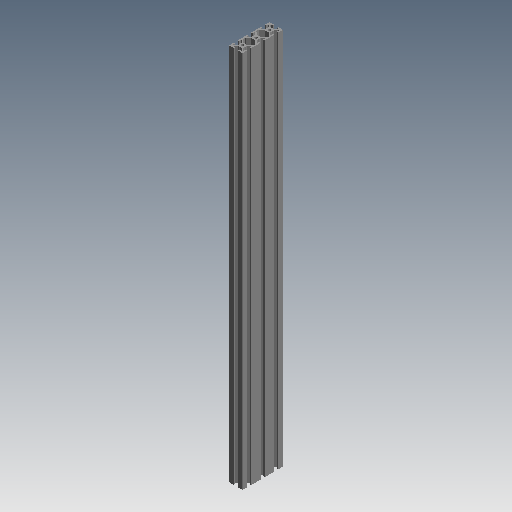
# Autodesk Inventor part: HFS5-2060-560
Saved by Autodesk Inventor 2020.1 (Build 241239000, 239)
## iProperties
Part Number: HFS5-2060-560
Material: 一般
Catalog Web Link: www.cadenas.de
Description: HFS5-2060, HFS5-2080, HFS5-4060, HFS5-4080, NFS5-2060, NFS5-2080, NFS5-4060, NFS5-4080-HFS5 Series Aluminum Extrusions 20mm Square -3 or more slots-
Vendor: MISUMI
Document SubType Name: Modeling
Designer: partserver
Manufacturer: MISUMI
Mass: 260.52 g
Surface Area: 2561.35 cm^2
Volume: 260.52 cm^3
Density: 1 g/cm^3
Appearance: PSOLRGB-175-175-175
Category: PARTsolutions
Company: MISUMI
PSOL_IDENT_0: {$CADENAS_DATA\23d-libs\misumi\metric\38_al_extrusions_blackets\5\hfs5_2060.prj},622 {VTYP=3D},{NB=H
PSOL_IDENT_1: FS5-2060-560},{LINA=HFS5-2060-560},{NN=HFS5-2060, HFS5-2080, HFS5-4060, HFS5-4080, NFS5-2060, NFS5-2
PSOL_IDENT_2: 080, NFS5-4060, NFS5-4080},{DATE=09.09.2019 15:28:27},{GEOMDATE=24.05.2018 01:50:00},{VERSION=},{LIN
PSOL_IDENT_3: EID=150},{WBVAR=L,ALT1,ALT2,ALT4,ALT5,CP5,DL5,DR5,ALT6,ALT9,ALT10,ALT11,HP6,NHL6,DL6,NHR6,DR6,ALT7,A
PSOL_IDENT_4: LT8,NH9,AH,BH,CH,DH,EH,NH10,AV,BV,CV,DV,EV,NH11,AP,BP,CP,DP,EP,ALT12,ALT13,Z,NH12,XA,XB,XC,XD,XE,NH1
PSOL_IDENT_5: 3,YA,YB,YC,YD,YE,ALT16,HP16,DL16,DR16,ALT17,HQ17,JLP,ALT18,HQ18,KLP,ALT20},{WBNUMERIC=L,NH9,AH,BH,CH
PSOL_IDENT_6: ,DH,EH,NH10,AV,BV,CV,DV,EV,NH11,AP,BP,CP,DP,EP,NH12,XA,XB,XC,XD,XE,NH13,YA,YB,YC,YD,YE,HQ17,JLP,HQ18
PSOL_IDENT_7: ,KLP}  {NB=HFS5-2060-560},{LINA=HFS5-2060-560},{KT=DUMMY},{PN=HFS5-2060-560},{TPS=HFS5-2060},{MAT=A6
PSOL_IDENT_8: N01SS-T5 Aluminum Alloy},{ST=Clear Anodize},{FRMW=20},{FRMH=60},{FRD=4.2},{L=560},{MASS=1.26},{SA=46
PSOL_IDENT_9: 4},{LX=1.97x10^4},{LY=15.98x10^4},{ALT1=},{M1=0},{DPL1=0},{DPR1=0},{ALT1PN=},{ALT2=},{ALT2ALG= '','w
PSOL_IDENT_10: /o End Tapping (Heli-Coil Insert)','LHP','with LHP (Tapping on the Left (Heli-Coil Insert))','RHP','
PSOL_IDENT_11: with RHP (Tapping on the Right (Heli-Coil Insert))','HPW','with HPW (Tapping on Both Ends (Heli-Coil
PSOL_IDENT_12: Insert))' },{M2=0},{DP2=0},{ALT2PN=},{ALT4=},{ALT4ALG= '', 'w/o SC (High Precision Cut)', 'SC', 'wi
PSOL_IDENT_13: th SC (High Precision Cut)' },{ALT4PN=},{ALT5=},{ALT5ALG= '','w/o 45 Degree Cut','1','with 45 Degree
PSOL_IDENT_14: Cut' },{CP5=},{CP5ALG= '','N/A' },{DL5=},{DL5ALG= '','N/A' },{DR5=},{DR5ALG= '','N/A' },{FRMLALT5=0
PSOL_IDENT_15: },{FRMRALT5=0},{ALT5PN=},{ALT6=},{ALT6ALG= '','w/o Fastening Location Wrench Access Hole Alterations'
PSOL_IDENT_16: ,'1','with Fastening Location Wrench Access Hole Alterations' },{ALT9=},{ALT9ALG= '','w/o Location S
PSOL_IDENT_17: pecified Wrench Access Hole Alteratons (Horizontal)','1','with Location Specified Wrench Access Hole
PSOL_IDENT_18: Alteratons (Horizontal)' },{ALT10=},{ALT10ALG= '','w/o Location Specified Wrench Access Hole Altera
PSOL_IDENT_19: tons (Vertical)','1','with Location Specified Wrench Access Hole Alteratons (Vertical)' },{ALT11=},{
PSOL_IDENT_20: ALT11ALG= '','w/o Location Specified Wrench Access Hole Alteratons (Crisscross)','1','with Location
PSOL_IDENT_21: Specified Wrench Access Hole Alteratons (Crisscross)' },{DD6=0.00},{DD6ALG=0},{HP6=},{HP6ALG= '','N/
PSOL_IDENT_22: A' },{NHL6=},{NHL6ALG= '','N/A' },{DL6=},{DL6ALG= '','N/A' },{NHR6=},{NHR6ALG= '','N/A' },{DR6=},{DR
PSOL_IDENT_23: 6ALG= '','N/A' },{DD6PN=},{HL6=0},{HL6D=0},{HR6=0},{HR6D=0},{J6=0},{J6D=0},{K6=0},{K6D=0},{ALT7=},{A
PSOL_IDENT_24: LT7ALG= '','N/A' },{ALT8=},{ALT8ALG= '','N/A' },{ALT678PN=},{NH9=0},{NH9MAX=5},{NH9ALG=[0]},{AH=0.0}
PSOL_IDENT_25: ,{AHMIN=7},{AHMAX=555},{AHALG=[0]},{BH=0.0},{BHMIN=2},{BHMAX=557},{BHALG=[0]},{CH=0.0},{CHMIN=2},{CH
PSOL_IDENT_26: MAX=559},{CHALG=[0]},{DH=0.0},{DHMIN=2},{DHMAX=561},{DHALG=[0]},{EH=0.0},{EHMIN=2},{EHMAX=553},{EHAL
PSOL_IDENT_27: G=[0]},{NH10=0},{NH10MAX=5},{NH10ALG=[0]},{AV=0.0},{AVMIN=7},{AVMAX=555},{AVALG=[0]},{BV=0.0},{BVMIN=
PSOL_IDENT_28: 2},{BVMAX=557},{BVALG=[0]},{CV=0.0},{CVMIN=2},{CVMAX=559},{CVALG=[0]},{DV=0.0},{DVMIN=2},{DVMAX=561}
PSOL_IDENT_29: ,{DVALG=[0]},{EV=0.0},{EVMIN=2},{EVMAX=553},{EVALG=[0]},{NH11=0},{NH11MAX=5},{NH11ALG=[0]},{AP=0.0},
PSOL_IDENT_30: {APMIN=7},{APMAX=555},{APALG=[0]},{BP=0.0},{BPMIN=2},{BPMAX=557},{BPALG=[0]},{CP=0.0},{CPMIN=2},{CPM
PSOL_IDENT_31: AX=559},{CPALG=[0]},{DP=0.0},{DPMIN=2},{DPMAX=561},{DPALG=[0]},{EP=0.0},{EPMIN=2},{EPMAX=553},{EPALG=
PSOL_IDENT_32: [0]},{ALT9PN=},{ALT10PN=},{ALT11PN=},{ALT91011PN=},{ALT12=},{ALT12ALG= '','w/o Counterbore Hole in S
PSOL_IDENT_33: pecified Position (Vertical)','1','with Counterbore Hole in Specified Position (Vertical)' },{ALT13=
PSOL_IDENT_34: },{ALT13ALG= '','w/o Counterbore Hole in Specified Position (Horizontal)','1','with Counterbore Hole
PSOL_IDENT_35: in Specified Position (Horizontal)' },{Z=},{ZALG= '','N/A' },{DD12=0.0},{DD112=0.0},{NH12=0},{NH12M
PSOL_IDENT_36: AX=5},{NH12ALG=[0]},{XA=0.0},{XAMIN=7},{XAMAX=555},{XAALG=[0]},{XB=0.0},{XBMIN=2},{XBMAX=557},{XBALG=
PSOL_IDENT_37: [0]},{XC=0.0},{XCMIN=2},{XCMAX=559},{XCALG=[0]},{XD=0.0},{XDMIN=2},{XDMAX=561},{XDALG=[0]},{XE=0.0},
PSOL_IDENT_38: {XEMIN=2},{XEMAX=553},{XEALG=[0]},{NH13=0},{NH13MAX=5},{NH13ALG=[0]},{YA=0.0},{YAMIN=7},{YAMAX=555},
PSOL_IDENT_39: {YAALG=[0]},{YB=0.0},{YBMIN=2},{YBMAX=557},{YBALG=[0]},{YC=0.0},{YCMIN=2},{YCMAX=559},{YCALG=[0]},{Y
PSOL_IDENT_40: D=0.0},{YDMIN=2},{YDMAX=561},{YDALG=[0]},{YE=0.0},{YEMIN=2},{YEMAX=553},{YEALG=[0]},{ALT12PN=},{ALT1
PSOL_IDENT_41: 3PN=},{ALT1213PN=},{ALT16=},{ALT16ALG= '','w/o M Type Hole Alteration','1','with M Type Hole Alterat
PSOL_IDENT_42: ion' },{HP16=},{HP16ALG= '','N/A' },{DL16=},{DL16ALG= '','N/A' },{DR16=},{DR16ALG= '','N/A' },{H116=
PSOL_IDENT_43: 0},{D16=0.0},{ALT16PN=},{ALT17=},{ALT17ALG= '','w/o L Type Hole Alteration (Top)','1','with L Type H
PSOL_IDENT_44: ole Alteration (Top)' },{HQ17=0},{HQ17ALG=0},{JLP=0},{JLPMIN=4.9},{JLPMAX=0},{JLPALG=[0]},{L17=0},{D
PSOL_IDENT_45: 17=0.0},{ALT17PN=},{ALT18=},{ALT18ALG= '','w/o L Type Hole Alteration (Bottom)','1','with L Type Hol
PSOL_IDENT_46: e Alteration (Bottom)' },{HQ18=0},{HQ18ALG=0},{KLP=0},{KLPMIN=4.9},{KLPMAX=0},{KLPALG=[0]},{L18=0},{
PSOL_IDENT_47: D18=0.0},{ALT18PN=},{ALT20=},{ALT20PN=},{ERRORALT01=OK},{ERRORALT02=OK},{ERRORALT05=OK},{ERRORALT060
PSOL_IDENT_48: 91=OK},{ERRORALT06092=OK},{ERRORALT06093=OK},{ERRORALT06094=OK},{ERRORALT06101=OK},{ERRORALT06102=OK
PSOL_IDENT_49: },{ERRORALT06103=OK},{ERRORALT06104=OK},{ERRORALT06111=OK},{ERRORALT06112=OK},{ERRORALT06113=OK},{ER
PSOL_IDENT_50: RORALT06114=OK},{ERRORALT06121=OK},{ERRORALT06122=OK},{ERRORALT06123=OK},{ERRORALT06124=OK},{ERRORAL
PSOL_IDENT_51: T06131=OK},{ERRORALT06132=OK},{ERRORALT06133=OK},{ERRORALT06134=OK},{ERRORALT0616=OK},{ERRORALT06171=
PSOL_IDENT_52: OK},{ERRORALT06172=OK},{ERRORALT06173=OK},{ERRORALT06181=OK},{ERRORALT06182=OK},{ERRORALT06183=OK},{
PSOL_IDENT_53: ERRORALT0911=OK},{ERRORALT0913=OK},{ERRORALT0916=OK},{ERRORALT0917=OK},{ERRORALT0918=OK},{ERRORALT10
PSOL_IDENT_54: 11=OK},{ERRORALT1012=OK},{ERRORALT1016=OK},{ERRORALT1017=OK},{ERRORALT1018=OK},{ERRORALT1112=OK},{ER
PSOL_IDENT_55: RORALT1113=OK},{ERRORALT1116=OK},{ERRORALT1117=OK},{ERRORALT1118=OK},{ERRORALT1216=OK},{ERRORALT1217=
PSOL_IDENT_56: OK},{ERRORALT1218=OK},{ERRORALT1316=OK},{ERRORALT1317=OK},{ERRORALT1318=OK},{ERRORALT1617=OK},{ERROR
PSOL_IDENT_57: ALT1618=OK},{ERRORPN=},{TFW=0}
NB: HFS5-2060-560
NN: HFS5-2060, HFS5-2080, HFS5-4060, HFS5-4080, NFS5-2060, NFS5-2080, NFS5-4060, NFS5-4080
NT: HFS5 Series Aluminum Extrusions 20mm Square -3 or more slots-
NBSYN: $PN.
LINA: HFS5-2060-560
CATALOG: Misumi
PN: HFS5-2060-560
TPS: HFS5-2060
MAT: A6N01SS-T5 Aluminum Alloy
ST: Clear Anodize
L: 560
MASS: 1.26
SA: 464
LX: 1.97x10^4
LY: 15.98x10^4
ALT1: w/o End Tapping
M1: 0
DPL1: 0
DPR1: 0
ALT2: w/o End Tapping (Heli-Coil Insert)
M2: 0
DP2: 0
ALT4: w/o SC (High Precision Cut)
ALT5: w/o 45 Degree Cut
CP5: N/A
DL5: N/A
DR5: N/A
ALT6: w/o Fastening Location Wrench Access Hole Alterations
ALT9: w/o Location Specified Wrench Access Hole Alteratons (Horizontal)
ALT10: w/o Location Specified Wrench Access Hole Alteratons (Vertical)
ALT11: w/o Location Specified Wrench Access Hole Alteratons (Crisscross)
DD6: 0
HP6: N/A
NHL6: N/A
DL6: N/A
NHR6: N/A
DR6: N/A
HL6D: 0
HR6D: 0
J6D: 0
K6D: 0
ALT7: N/A
ALT8: N/A
NH9: 0
AH: 0
BH: 0
CH: 0
DH: 0
EH: 0
NH10: 0
AV: 0
BV: 0
CV: 0
DV: 0
EV: 0
NH11: 0
AP: 0
BP: 0
CP: 0
DP: 0
EP: 0
ALT12: w/o Counterbore Hole in Specified Position (Vertical)
ALT13: w/o Counterbore Hole in Specified Position (Horizontal)
Z: N/A
DD12: 0
DD112: 0
NH12: 0
XA: 0
XB: 0
XC: 0
XD: 0
XE: 0
NH13: 0
YA: 0
YB: 0
YC: 0
YD: 0
YE: 0
ALT16: w/o M Type Hole Alteration
HP16: N/A
DL16: N/A
DR16: N/A
H116: 0
D16: 0
ALT17: w/o L Type Hole Alteration (Top)
HQ17: 0
JLP: 0
D17: 0
ALT18: w/o L Type Hole Alteration (Bottom)
HQ18: 0
KLP: 0
D18: 0
ALT20: w/o CW (End Face C Chamfering)
SUPPLIER: MISUMI
ARTICLENO: HFS5-2060-560
BOMINFO: HFS5-2060-560
CREATOR: CADENAS GmbH
Title: HFS5-2060-560
Author: Cadenas PARTsolutions
Comments: HFS5 Series Aluminum Extrusions 20mm Square -3 or more slots-
Autodesk Inventor part; units mm, degrees
ref_plane "YZ Plane" through (0, 0, 0) normal (1, 0, 0) x (0, 1, 0)
ref_plane "XZ Plane" through (0, 0, 0) normal (0, 1, 0) x (-1, 0, 0)
ref_plane "XY Plane" through (0, 0, 0) normal (0, 0, 1) x (1, 0, 0)
sketch "Sketch_100" plane through (0, 0, 0) normal (0, 0, 1) x (1, 0, 0)
  line L0 (-10, -17) -> (-8, -17)
  line L1 (-8, -17) -> (-8, -14)
  line L2 (-8, -14) -> (-7.0607, -14)
  line L3 (-7.0607, -14) -> (-4, -17.0607)
  line L4 (-4, -17.0607) -> (-4, -19.4804)
  line L5 (-4, -19.4804) -> (-3.7, -20)
  line L6 (-3.7, -20) -> (-4, -20.5196)
  line L7 (-4, -20.5196) -> (-4, -22.9393)
  line L8 (-4, -22.9393) -> (-7.0607, -26)
  line L9 (-7.0607, -26) -> (-8, -26)
  line L10 (-8, -26) -> (-8, -23)
  line L11 (-8, -23) -> (-10, -23)
  line L12 (-10, -23) -> (-10, -29)
  arc A0 (-10, -29) -> (-9, -30) centre (-9, -29) ccw
  line L13 (-9, -30) -> (-3, -30)
  line L14 (-3, -30) -> (-3, -28)
  line L15 (-3, -28) -> (-6, -28)
  line L16 (-6, -28) -> (-6, -27.0607)
  line L17 (-6, -27.0607) -> (-2.9393, -24)
  line L18 (-2.9393, -24) -> (-0.5196, -24)
  line L19 (-0.5196, -24) -> (0, -23.7)
  line L20 (0, -23.7) -> (0.5196, -24)
  line L21 (0.5196, -24) -> (2.9393, -24)
  line L22 (2.9393, -24) -> (6, -27.0607)
  line L23 (6, -27.0607) -> (6, -28)
  line L24 (6, -28) -> (3, -28)
  line L25 (3, -28) -> (3, -30)
  line L26 (3, -30) -> (9, -30)
  arc A1 (9, -30) -> (10, -29) centre (9, -29) ccw
  line L27 (10, -29) -> (10, -23)
  line L28 (10, -23) -> (8, -23)
  line L29 (8, -23) -> (8, -26)
  line L30 (8, -26) -> (7.0607, -26)
  line L31 (7.0607, -26) -> (4, -22.9393)
  line L32 (4, -22.9393) -> (4, -20.5196)
  line L33 (4, -20.5196) -> (3.7, -20)
  line L34 (3.7, -20) -> (4, -19.4804)
  line L35 (4, -19.4804) -> (4, -17.0607)
  line L36 (4, -17.0607) -> (7.0607, -14)
  line L37 (7.0607, -14) -> (8, -14)
  line L38 (8, -14) -> (8, -17)
  line L39 (8, -17) -> (10, -17)
  line L40 (10, -17) -> (10, -3)
  line L41 (10, -3) -> (8, -3)
  line L42 (8, -3) -> (8, -6)
  line L43 (8, -6) -> (7.0607, -6)
  line L44 (7.0607, -6) -> (4, -2.9393)
  line L45 (4, -2.9393) -> (4, -0.5196)
  line L46 (4, -0.5196) -> (3.7, 0)
  line L47 (3.7, 0) -> (4, 0.5196)
  line L48 (4, 0.5196) -> (4, 2.9393)
  line L49 (4, 2.9393) -> (7.0607, 6)
  line L50 (7.0607, 6) -> (8, 6)
  line L51 (8, 6) -> (8, 3)
  line L52 (8, 3) -> (10, 3)
  line L53 (10, 3) -> (10, 17)
  line L54 (10, 17) -> (8, 17)
  line L55 (8, 17) -> (8, 14)
  line L56 (8, 14) -> (7.0607, 14)
  line L57 (7.0607, 14) -> (4, 17.0607)
  line L58 (4, 17.0607) -> (4, 19.4804)
  line L59 (4, 19.4804) -> (3.7, 20)
  line L60 (3.7, 20) -> (4, 20.5196)
  line L61 (4, 20.5196) -> (4, 22.9393)
  line L62 (4, 22.9393) -> (7.0607, 26)
  line L63 (7.0607, 26) -> (8, 26)
  line L64 (8, 26) -> (8, 23)
  line L65 (8, 23) -> (10, 23)
  line L66 (10, 23) -> (10, 29)
  arc A2 (10, 29) -> (9, 30) centre (9, 29) ccw
  line L67 (9, 30) -> (3, 30)
  line L68 (3, 30) -> (3, 28)
  line L69 (3, 28) -> (6, 28)
  line L70 (6, 28) -> (6, 27.0607)
  line L71 (6, 27.0607) -> (2.9393, 24)
  line L72 (2.9393, 24) -> (0.5196, 24)
  line L73 (0.5196, 24) -> (0, 23.7)
  line L74 (0, 23.7) -> (-0.5196, 24)
  line L75 (-0.5196, 24) -> (-2.9393, 24)
  line L76 (-2.9393, 24) -> (-6, 27.0607)
  line L77 (-6, 27.0607) -> (-6, 28)
  line L78 (-6, 28) -> (-3, 28)
  line L79 (-3, 28) -> (-3, 30)
  line L80 (-3, 30) -> (-9, 30)
  arc A3 (-9, 30) -> (-10, 29) centre (-9, 29) ccw
  line L81 (-10, 29) -> (-10, 23)
  line L82 (-10, 23) -> (-8, 23)
  line L83 (-8, 23) -> (-8, 26)
  line L84 (-8, 26) -> (-7.0607, 26)
  line L85 (-7.0607, 26) -> (-4, 22.9393)
  line L86 (-4, 22.9393) -> (-4, 20.5196)
  line L87 (-4, 20.5196) -> (-3.7, 20)
  line L88 (-3.7, 20) -> (-4, 19.4804)
  line L89 (-4, 19.4804) -> (-4, 17.0607)
  line L90 (-4, 17.0607) -> (-7.0607, 14)
  line L91 (-7.0607, 14) -> (-8, 14)
  line L92 (-8, 14) -> (-8, 17)
  line L93 (-8, 17) -> (-10, 17)
  line L94 (-10, 17) -> (-10, 3)
  line L95 (-10, 3) -> (-8, 3)
  line L96 (-8, 3) -> (-8, 6)
  line L97 (-8, 6) -> (-7.0607, 6)
  line L98 (-7.0607, 6) -> (-4, 2.9393)
  line L99 (-4, 2.9393) -> (-4, 0.5196)
  line L100 (-4, 0.5196) -> (-3.7, 0)
  line L101 (-3.7, 0) -> (-4, -0.5196)
  line L102 (-4, -0.5196) -> (-4, -2.9393)
  line L103 (-4, -2.9393) -> (-7.0607, -6)
  line L104 (-7.0607, -6) -> (-8, -6)
  line L105 (-8, -6) -> (-8, -3)
  line L106 (-8, -3) -> (-10, -3)
  line L107 (-10, -3) -> (-10, -17)
  line L108 (-8, 8) -> (-6.9393, 8)
  line L109 (-6.9393, 8) -> (-2.9393, 4)
  line L110 (-2.9393, 4) -> (2.9393, 4)
  line L111 (2.9393, 4) -> (6.9393, 8)
  line L112 (6.9393, 8) -> (8, 8)
  line L113 (8, 8) -> (8, 12)
  line L114 (8, 12) -> (6.9393, 12)
  line L115 (6.9393, 12) -> (2.9393, 16)
  line L116 (2.9393, 16) -> (-2.9393, 16)
  line L117 (-2.9393, 16) -> (-6.9393, 12)
  line L118 (-6.9393, 12) -> (-8, 12)
  line L119 (-8, 12) -> (-8, 8)
  line L120 (-8, -8) -> (-8, -12)
  line L121 (-8, -12) -> (-6.9393, -12)
  line L122 (-6.9393, -12) -> (-2.9393, -16)
  line L123 (-2.9393, -16) -> (2.9393, -16)
  line L124 (2.9393, -16) -> (6.9393, -12)
  line L125 (6.9393, -12) -> (8, -12)
  line L126 (8, -12) -> (8, -8)
  line L127 (8, -8) -> (6.9393, -8)
  line L128 (6.9393, -8) -> (2.9393, -4)
  line L129 (2.9393, -4) -> (-2.9393, -4)
  line L130 (-2.9393, -4) -> (-6.9393, -8)
  line L131 (-6.9393, -8) -> (-8, -8)
  constraints: 264 end point, 8 point on circle, 4 centre point
extrude "Extrusion1" add sketch "Sketch_100" against normal blind 560
sketch "Sketch2" plane through (0, 0, 0) normal (0, 0, 1) x (1, 0, 0)
  point P0 (0, 20)
hole "Hole1" at (0, 20, 0) direction (0, 0, -1) diameter 4.2 depth 560
pattern_linear "Rectangular Pattern1" count 3 spacing 20 along (0, -1, 0) of "Hole1"
body "Solid1"
